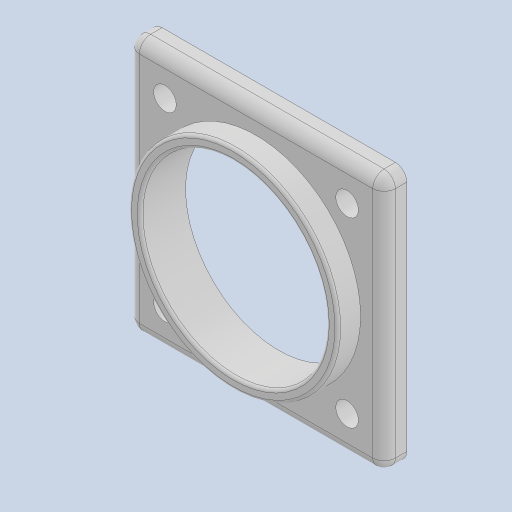
# Autodesk Inventor part: cage_outside_01
Saved by Autodesk Inventor 2024.4 (Build 284460000, 460)
## iProperties
Created: 2026-03-25
Part Number: cage_outside_01
Material: Generic
Document SubType Name: Modeling
Designer: tooles01
Density: 1 g/cm^3
Appearance: Default
Author: tooles01
Autodesk Inventor part; units mm, degrees
ref_plane "YZ Plane" through (0, 0, 0) normal (1, 0, 0) x (0, 1, 0)
ref_plane "XZ Plane" through (0, 0, 0) normal (0, 1, 0) x (-1, 0, 0)
ref_plane "XY Plane" through (0, 0, 0) normal (0, 0, 1) x (1, 0, 0)
derived "cage_inside_01.ipt"
sketch "Sketch1: base" plane through (0, 0, 0) normal (0, 0, 1) x (1, 0, 0)
  line L0 (-22.9459, 27.4044) -> (22.0541, 27.4044)
  line L1 (22.0541, 27.4044) -> (22.0541, -17.5956)
  line L2 (22.0541, -17.5956) -> (-22.9459, -17.5956)
  line L3 (-22.9459, -17.5956) -> (-22.9459, 27.4044)
  circle A0 centre (-0.4459, 4.9044) radius 16.375
  line L4 (-16.4459, 20.9044) -> (15.5541, 20.9044) construction
  line L5 (15.5541, 20.9044) -> (15.5541, -11.0956) construction
  line L6 (15.5541, -11.0956) -> (-16.4459, -11.0956) construction
  line L7 (-16.4459, -11.0956) -> (-16.4459, 20.9044) construction
  circle A1 centre (-0.4459, 4.9044) radius 14.875
  circle A2 centre (15.5541, 20.9044) radius 1.8 construction
  circle A3 centre (15.5541, 20.9044) radius 3.25 construction
  point P0 (0, 0)
  point P1 (22.0541, 4.9044)
  point P2 (-0.4459, 27.4044)
  point P3 (-0.4459, 20.9044)
  point P4 (-16.4459, 4.9044)
extrude "Ex1: base" add sketch "Sketch1: base" along normal blind 4 contours L0 L1 L2 L3
hole "Hole1: M3 inserts" at (-16.4459, 20.9044, 0) at (15.5541, 20.9044, 0) at (-16.4459, -11.0956, 0) at (15.5541, -11.0956, 0) direction (0, 0, 1) diameter 4 end through all
fillet "Fillet1" radius 2 8 edges at (-0.4459, 27.4044, 4) (22.0541, 4.9044, 4) (-22.9459, 4.9044, 4) (-0.4459, -17.5956, 4) (22.0541, -17.5956, 2) (22.0541, 27.4044, 2) (-22.9459, 27.4044, 2) (-22.9459, -17.5956, 2)
sketch "Sketch2: tube connection" plane through (0, 0, 0) normal (0, 0, 1) x (1, 0, 0)
  circle A0 centre (-0.4459, 4.9044) radius 16.375 projected
  circle A1 centre (-0.4459, 4.9044) radius 18.375
  point P0 (0, 0)
  dimension "d12" = 2
  constraints: 1 centre point, 1 coincident
  measures "d12" radial gap between concentric circles of A0 A1
extrude "Ex2: tube fit" add sketch "Sketch2: tube connection" along normal blind 4 from surface at 4
fillet "Fillet2" radius 0.5 2 edges at (-16.8209, 4.9044, 8) (-18.8209, 4.9044, 8)
body "Solid1"
